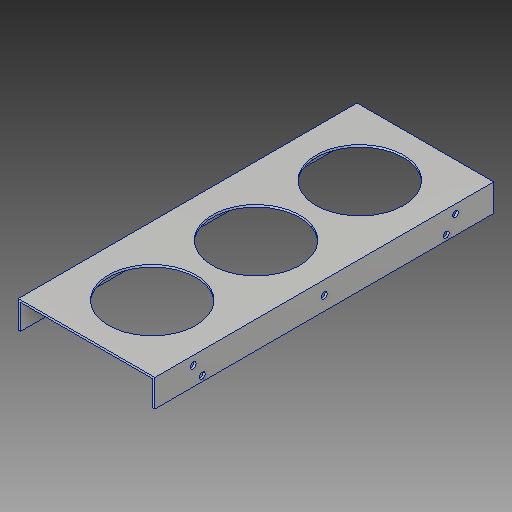
# Autodesk Inventor part: Mottor Protection Piece
Saved by Autodesk Inventor 2019.4 (Build 234330000, 330)
## iProperties
Created: 2019-11-02
Part Number: Mottor Protection Piece
Material: Aluminum 6061
Document SubType Name: Modeling
Designer: admin
Density: 2.7 g/cm^3
Appearance: Aluminum - Flat
Mass: 203.541 g
Surface Area: 791.631 cm^2
Volume: 75.3855 cm^3
Author: admin
Autodesk Inventor part; units mm, degrees
ref_plane "YZ Plane" through (0, 0, 0) normal (1, 0, 0) x (0, 1, 0)
ref_plane "XZ Plane" through (0, 0, 0) normal (0, 1, 0) x (-1, 0, 0)
ref_plane "XY Plane" through (0, 0, 0) normal (0, 0, 1) x (1, 0, 0)
sketch "Sketch1" plane through (0, 0, 0) normal (0, 0, 1) x (1, 0, 0)
  line L0 (0, 0) -> (0, 25)
  line L1 (0, 25) -> (125, 25)
  line L2 (125, 25) -> (125, 0)
  line L3 (123, 0) -> (123, 23)
  line L4 (123, 23) -> (2, 23)
  line L5 (2, 23) -> (2, 0)
  line L6 (0, 0) -> (2, 0)
  line L7 (123, 0) -> (125, 0)
  dimension "d0" = 25
  dimension "d1" = 125
  dimension "d2" = 25
  dimension "d3" = 2
  constraints: 16 end point, 4 perpendicular, 1 collinear, 1 horizontal, 1 vertical, 2 other
  measures "d0" distance of L0.start L0.end
  measures "d1" distance of L0.end L1.end
  measures "d2" distance of L1.end L2.end
  measures "d3" distance between parallel lines of L1 L4
extrude "Extrusion1" add sketch "Sketch1" along normal mid plane 310
sketch "Sketch2" plane through (125, 0, 155) normal (1, 0, 0) x (0, 0, -1)
  line L0 (-37.205, -32.4182) -> (-17.0936, -51.4126) projected
  arc A0 (-19.5275, -56.5702) -> (-17.0936, -51.4126) centre (-19.1534, -53.5936) ccw projected
  line L1 (-19.5275, -56.5702) -> (-48.3213, -52.9518) projected
  arc A1 (-48.3213, -52.9518) -> (-53.9507, -41.6522) centre (-69.9997, -56.6998) ccw projected
  line L2 (-53.9507, -41.6522) -> (-47.6036, -32.0405) projected
  arc A2 (-47.6036, -32.0405) -> (-37.205, -32.4182) centre (-41.913, -18.7038) ccw projected
  line L3 (-75.1262, -21.5392) -> (-58.4114, -21.5392) projected
  arc A3 (-55.5831, -23.5388) -> (-58.4114, -21.5392) centre (-58.4114, -24.5392) ccw projected
  arc A4 (-55.5831, -23.5388) -> (-54.0496, -26.638) centre (-41.913, -18.7038) ccw projected
  arc A5 (-54.1934, -30.1224) -> (-54.0496, -26.638) centre (-56.5606, -28.2795) ccw projected
  line L4 (-54.1934, -30.1224) -> (-58.2717, -35.3612) projected
  arc A6 (-61.7623, -36.3002) -> (-58.2717, -35.3612) centre (-60.639, -33.5184) ccw projected
  arc A7 (-61.7623, -36.3002) -> (-91.7666, -59.8942) centre (-69.9997, -56.6998) ccw projected
  arc A8 (-91.9336, -61.4039) -> (-91.7666, -59.8942) centre (-94.7348, -60.3298) ccw projected
  arc A9 (-94.9246, -58.6363) -> (-91.9336, -61.4039) centre (-91.9336, -58.4039) ccw projected
  arc A10 (-90.8616, -42.9236) -> (-94.9246, -58.6363) centre (-69.9997, -56.6998) ccw projected
  line L5 (-90.8616, -42.9236) -> (-77.6297, -22.886) projected
  arc A11 (-75.1262, -21.5392) -> (-77.6297, -22.886) centre (-75.1262, -24.5392) ccw projected
  line L6 (14.2226, -42.1262) -> (14.481, -34.3473) projected
  arc A12 (16.1692, -31.7481) -> (14.481, -34.3473) centre (17.4793, -34.4469) ccw projected
  arc A13 (16.1692, -31.7481) -> (22.7187, -25.3606) centre (9.837, -18.7038) ccw projected
  arc A14 (25.3838, -23.7379) -> (22.7187, -25.3606) centre (25.3838, -26.7379) ccw projected
  line L7 (25.3838, -23.7379) -> (32.9823, -23.7379) projected
  arc A15 (35.8164, -27.7217) -> (32.9823, -23.7379) centre (32.9823, -26.7379) ccw projected
  arc A16 (20.9479, -43.8593) -> (35.8164, -27.7217) centre (9.837, -18.7038) ccw projected
  line L8 (20.9479, -43.8593) -> (18.4331, -44.97) projected
  arc A17 (14.2226, -42.1262) -> (18.4331, -44.97) centre (17.221, -42.2258) ccw projected
  arc A18 (-52.6191, -70.1873) -> (-49.4307, -64.5046) centre (-69.9997, -56.6998) ccw projected
  arc A19 (-46.238, -62.5941) -> (-49.4307, -64.5046) centre (-46.6258, -65.5689) ccw projected
  line L9 (-46.238, -62.5941) -> (-37.7469, -63.701) projected
  arc A20 (-36.9226, -69.42) -> (-37.7469, -63.701) centre (-38.1347, -66.6758) ccw projected
  line L10 (-36.9226, -69.42) -> (-49.0369, -74.7708) projected
  arc A21 (-52.6191, -70.1873) -> (-49.0369, -74.7708) centre (-50.249, -72.0265) ccw projected
  arc A22 (-86.9907, -75.0384) -> (-80.1014, -79.568) centre (-69.9997, -56.6998) ccw projected
  arc A23 (-86.7344, -71.903) -> (-86.9907, -75.0384) centre (-85.6314, -73.5713) ccw projected
  arc A24 (-85.3399, -72.4694) -> (-86.7344, -71.903) centre (-86.7344, -73.903) ccw projected
  arc A25 (-85.3399, -72.4694) -> (-80.2891, -76.1453) centre (-69.9997, -56.6998) ccw projected
  arc A26 (-80.1014, -79.568) -> (-80.2891, -76.1453) centre (-81.2245, -77.9131) ccw projected
  line L11 (14.545, -2.9927) -> (14.545, 4.5521) projected
  arc A27 (18.4889, 7.3998) -> (14.545, 4.5521) centre (17.545, 4.5521) ccw projected
  arc A28 (35.8164, -9.6858) -> (18.4889, 7.3998) centre (9.837, -18.7038) ccw projected
  arc A29 (32.9823, -13.6696) -> (35.8164, -9.6858) centre (32.9823, -10.6696) ccw projected
  line L12 (32.9823, -13.6696) -> (25.3838, -13.6696) projected
  arc A30 (22.7187, -12.0469) -> (25.3838, -13.6696) centre (25.3838, -10.6696) ccw projected
  arc A31 (22.7187, -12.0469) -> (16.2237, -5.6861) centre (9.837, -18.7038) ccw projected
  arc A32 (14.545, -2.9927) -> (16.2237, -5.6861) centre (17.545, -2.9927) ccw projected
  line L13 (-41.913, 8.7962) -> (-41.4149, 8.7962) projected
  arc A33 (-38.601, 4.7561) -> (-41.4149, 8.7962) centre (-41.4149, 5.7962) ccw projected
  line L14 (-38.601, 4.7561) -> (-41.237, -2.375) projected
  arc A34 (-43.6844, -4.3124) -> (-41.237, -2.375) centre (-44.0509, -1.3349) ccw projected
  arc A35 (-43.6844, -4.3124) -> (-55.5831, -13.8687) centre (-41.913, -18.7038) ccw projected
  arc A36 (-58.4114, -15.8684) -> (-55.5831, -13.8687) centre (-58.4114, -12.8684) ccw projected
  line L15 (-58.4114, -15.8684) -> (-67.4194, -15.8684) projected
  arc A37 (-69.9228, -11.2152) -> (-67.4194, -15.8684) centre (-67.4194, -12.8684) ccw projected
  line L16 (-69.9228, -11.2152) -> (-64.861, -3.5499) projected
  arc A38 (-41.913, 8.7962) -> (-64.861, -3.5499) centre (-41.913, -18.7038) ccw projected
  line L17 (-27.9232, -22.5166) -> (-4.1527, -22.5166) projected
  arc A39 (-4.1527, -22.5166) -> (3.5036, -31.7475) centre (9.837, -18.7038) ccw projected
  arc A40 (5.1099, -35.1484) -> (3.5036, -31.7475) centre (2.1933, -34.4462) ccw projected
  line L18 (5.1099, -35.1484) -> (1.9297, -48.3572) projected
  arc A41 (-2.7527, -50.0803) -> (1.9297, -48.3572) centre (-0.9869, -47.6549) ccw projected
  line L19 (-2.7527, -50.0803) -> (-31.7052, -29.0019) projected
  arc A42 (-31.7052, -29.0019) -> (-27.9232, -22.5166) centre (-41.913, -18.7038) ccw projected
  line L20 (-6.2824, -14.891) -> (-25.7935, -14.891) projected
  arc A43 (-28.5569, -13.0589) -> (-25.7935, -14.891) centre (-25.7935, -11.891) ccw projected
  arc A44 (-28.5569, -13.0589) -> (-34.5765, -6.1967) centre (-41.913, -18.7038) ccw projected
  arc A45 (-35.7016, -2.1898) -> (-34.5765, -6.1967) centre (-33.0586, -3.6091) ccw projected
  line L21 (-35.7016, -2.1898) -> (-30.651, 7.2155) projected
  arc A46 (-28.008, 8.7962) -> (-30.651, 7.2155) centre (-28.008, 5.7962) ccw projected
  line L22 (-28.008, 8.7962) -> (-0.2731, 8.7962) projected
  arc A47 (2.7269, 5.7962) -> (-0.2731, 8.7962) centre (-0.2731, 5.7962) ccw projected
  line L23 (2.7269, 5.7962) -> (2.7269, -4.4197) projected
  arc A48 (1.46, -6.8684) -> (2.7269, -4.4197) centre (-0.2731, -4.4197) ccw projected
  arc A49 (1.46, -6.8684) -> (-3.5191, -13.0589) centre (9.837, -18.7038) ccw projected
  arc A50 (-6.2824, -14.891) -> (-3.5191, -13.0589) centre (-6.2824, -11.891) ccw projected
  circle A51 centre (-81.913, -5.781) radius 2.75 projected
  circle A52 centre (7.837, -58.4172) radius 2.75 projected
  circle A53 centre (-19.913, 17.776) radius 2.75 projected
  circle A54 centre (-109.9997, -47.6996) radius 2.75 projected
  circle A55 centre (43.4223, 4.8129) radius 2.75 projected
  line L24 (-25.906, 18.0659) -> (-40.1014, 18.7524) projected
  arc A56 (-40.1014, 18.7524) -> (-73.2057, 1.9606) centre (-41.913, -18.7038) ccw projected
  line L25 (-73.2057, 1.9606) -> (-74.4501, 0.0761) projected
  arc A57 (-78.6067, -0.7742) -> (-82.3668, 0.2018) centre (-81.913, -5.781) ccw projected
  line L26 (-85.6456, -16.8777) -> (-99.2063, -37.4131) projected
  arc A58 (-99.2063, -37.4131) -> (-100.1023, -38.8439) centre (-69.9997, -56.6998) ccw projected
  arc A59 (-113.4192, -52.6298) -> (-109.9997, -53.6996) centre (-109.9997, -47.6996) ccw projected
  line L27 (-109.9997, -53.6996) -> (-107.9997, -53.6996) projected
  arc A60 (-104.9997, -56.6996) -> (-54.959, -88.3032) centre (-69.9997, -56.6998) ccw projected
  line L28 (-54.959, -88.3032) -> (2.4193, -60.9957) projected
  arc A61 (2.4193, -60.9957) -> (13.2548, -55.8388) centre (7.837, -58.4172) ccw projected
  line L29 (13.2548, -55.8388) -> (24.8778, -50.3072) projected
  arc A62 (24.8778, -50.3072) -> (42.845, -7.0644) centre (9.837, -18.7038) ccw projected
  line L30 (42.845, -7.0644) -> (48.4494, 1.5375) projected
  arc A63 (48.4494, 1.5375) -> (42.0639, 10.6571) centre (43.4223, 4.8129) ccw projected
  line L31 (42.0639, 10.6571) -> (32.0639, 8.3327) projected
  arc A64 (32.0639, 8.3327) -> (11.5279, 16.2554) centre (9.837, -18.7038) ccw projected
  line L32 (11.5279, 16.2554) -> (-13.92, 17.4862) projected
  arc A65 (-13.92, 17.4862) -> (-25.906, 18.0659) centre (-19.913, 17.776) ccw projected
  circle A66 centre (-69.9997, -56.6998) radius 12 projected
  circle A67 centre (-41.913, -18.7038) radius 9.5 projected
  circle A68 centre (9.837, -18.7038) radius 9.5 projected
  circle A69 centre (35, 17) radius 2.75
  circle A70 centre (155, 12.5) radius 2.75
  line L33 (155, 0) -> (155, 25)
  line L34 (0, 25) -> (310, 25) projected
  line L35 (0, 0) -> (0, 25) projected
  circle A71 centre (266.5777, 4.8129) radius 2.75
  circle A72 centre (275, 17) radius 2.75
  circle A73 centre (155, 12.5) radius 2.75
  circle A74 centre (-106.7656, -26.4398) radius 1.65 projected
  arc A75 (-104.9997, -56.6996) -> (-107.9997, -53.6996) centre (-107.9997, -56.6996) ccw projected
  arc A76 (-78.6067, -0.7742) -> (-74.4501, 0.0761) centre (-76.9535, 1.7293) ccw projected
  line L36 (-82.3668, 0.2018) -> (-122.8325, -2.8676) projected
  arc A77 (-122.8325, -2.8676) -> (-132.7182, -39.2443) centre (-121.3198, -22.8103) ccw projected
  line L37 (-132.7182, -39.2443) -> (-113.4192, -52.6298) projected
  circle A78 centre (-131.7402, -33.5999) radius 1.65 projected
  circle A79 centre (-121.3198, -22.8103) radius 10.5 projected
  circle A80 centre (-125.4537, -8.3911) radius 1.65 projected
  line L38 (-104.3923, -39.7785) -> (-104.8988, -39.4272) projected
  arc A81 (-105.5539, -35.1162) -> (-104.8988, -39.4272) centre (-103.189, -36.9621) ccw projected
  arc A82 (-105.5539, -35.1162) -> (-102.1972, -16.9514) centre (-121.3198, -22.8103) ccw projected
  arc A83 (-99.5557, -13.0811) -> (-102.1972, -16.9514) centre (-99.3288, -16.0725) ccw projected
  line L39 (-99.5557, -13.0811) -> (-88.3759, -12.2331) projected
  arc A84 (-85.6456, -16.8777) -> (-88.3759, -12.2331) centre (-88.149, -15.2245) ccw projected
  arc A85 (-104.3923, -39.7785) -> (-100.1023, -38.8439) centre (-102.6826, -37.3134) ccw projected
  point P0 (-69.9997, -56.6998)
  point P1 (-69.9997, -56.6998)
  point P2 (-69.9997, -56.6998)
  point P3 (-69.9997, -56.6998)
  point P4 (-107.9997, -56.6996)
  point P5 (-102.6826, -37.3134)
  dimension "d6" = 5.5
  dimension "d7" = 5.5
  dimension "d8" = 8
  dimension "d9" = 12.5
  dimension "d10" = 35
  constraints: 5 centre point, 2 end point, 2 midpoint, 2 symmetric about line, 3 other
  measures "d6" diameter of A69
  measures "d7" diameter of A70
  measures "d8" distance from line of L34 A69.centre
  measures "d9" distance from line of L34 A70.centre
  measures "d10" distance from line of L35 A69.centre
extrude "Extrusion2" cut sketch "Sketch2" against normal blind 205.75 contours A55 | A69 | A70 L33 | L33 A70 | A71 | A72
sketch "Sketch3" plane through (0, 25, 155) normal (0, 1, 0) x (1, 0, 0)
  circle A0 centre (62.5, 60) radius 40
  line L0 (125, 0) -> (125, 310) projected
  line L1 (125, 0) -> (0, 0) projected
  circle A1 centre (62.5, 250) radius 40
  line L2 (0, 310) -> (125, 310) projected
  circle A2 centre (62.5, 155) radius 40
  point P0 (0, 155)
  dimension "d13" = 80
  dimension "d14" = 62.5
  dimension "d15" = 60
  dimension "d16" = 80
  dimension "d17" = 62.5
  dimension "d18" = 60
  dimension "d19" = 80
  dimension "d20" = 62.5
  dimension "d21" = 155
  constraints: 3 centre point
  measures "d13" diameter of A0
  measures "d14" distance from line of L0 A0.centre
  measures "d15" distance from line of L1 A0.centre
  measures "d16" diameter of A1
  measures "d17" distance from line of L0 A1.centre
  measures "d18" distance from line of L2 A1.centre
  measures "d19" diameter of A2
  measures "d20" distance from line of L0 A2.centre
  measures "d21" distance from line of L2 A2.centre
extrude "Extrusion3" cut sketch "Sketch3" against normal blind 10
body "Solid1"
